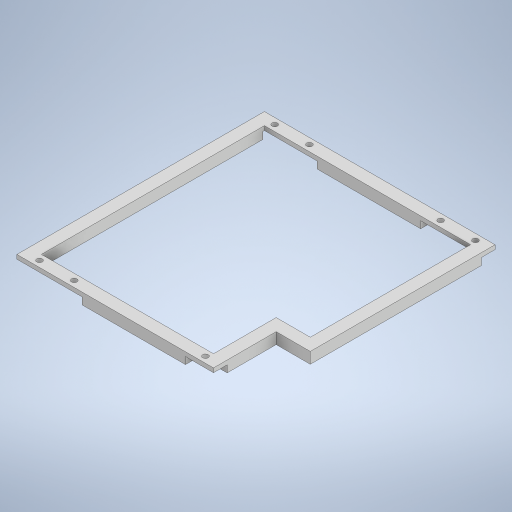
# Autodesk Inventor part: Base PCB
Saved by Autodesk Inventor 2024 (Build 280153000, 153)
## iProperties
Created: 2023-06-25
Part Number: Base PCB
Material: Genérico
Document SubType Name: Modeling
Designer: sergi
Density: 1 g/cm^3
Appearance: Valor por defecto
Author: sergi
Autodesk Inventor part; units mm, degrees
ref_plane "YZ Plane" through (0, 0, 0) normal (1, 0, 0) x (0, 1, 0)
ref_plane "XZ Plane" through (0, 0, 0) normal (0, 1, 0) x (-1, 0, 0)
ref_plane "XY Plane" through (0, 0, 0) normal (0, 0, 1) x (1, 0, 0)
sketch "Boceto1" plane through (0, 0, 0) normal (0, 1, 0) x (-1, 0, 0)
  line L0 (0, 0) -> (262.4667, 0) construction
  line L1 (262.4667, 0) -> (262.4667, -371.2633) construction
  line L2 (262.4667, -371.2633) -> (0, -371.2633) construction
  line L3 (0, -371.2633) -> (0, 0) construction
  line L4 (167.9771, -4.7349) -> (167.9771, -13.5349)
  line L5 (167.9771, -13.5349) -> (2.3545, -13.5349)
  line L6 (2.3545, -13.5349) -> (2.3545, -4.7349)
  line L7 (2.3545, -4.7349) -> (167.9771, -4.7349)
  line L8 (143.5689, -182.4039) -> (2.3545, -182.4039)
  line L9 (2.3545, -182.4039) -> (2.3545, -173.6039)
  line L10 (2.3545, -173.6039) -> (167.9771, -173.6039)
  line L11 (167.9771, -173.6039) -> (167.9771, -182.4039)
  circle A0 centre (156.1475, -9.1349) radius 2
  circle A1 centre (131.2333, -9.1349) radius 2
  circle A2 centre (12.066, -9.1349) radius 2
  line L12 (167.9771, -173.6039) -> (167.9771, -182.4039)
  line L13 (167.9771, -182.4039) -> (2.3545, -182.4039)
  line L14 (2.3545, -182.4039) -> (2.3545, -173.6039)
  line L15 (2.3545, -173.6039) -> (167.9771, -173.6039)
  circle A3 centre (131.2333, -178.0039) radius 2
  circle A4 centre (12.066, -178.0039) radius 2
  line L16 (167.9771, -13.5349) -> (167.9771, -182.4039)
  line L17 (2.3545, -13.4261) -> (2.3545, -174.0455)
  line L18 (11.1545, -13.4261) -> (11.1545, -174.0455)
  line L19 (159.1771, -13.5349) -> (159.1771, -182.4039)
  line L20 (26.8486, -4.7349) -> (26.8486, -49.7349)
  line L21 (26.8486, -49.7349) -> (2.3545, -49.7349)
  line L22 (35.6486, -4.7349) -> (35.6486, -58.5349)
  line L23 (35.6486, -58.5349) -> (2.3545, -58.5349)
  point P0 (11.1545, -173.6039)
  point P1 (11.1545, -13.5349)
  point P2 (159.1771, -173.6039)
  point P3 (11.1545, -58.5349)
  point P4 (35.6486, -13.5349)
  dimension "d2" = 8.8
  dimension "d3" = 8.8
  dimension "d5" = 8.8
  dimension "d6" = 8.8
  dimension "d8" = 4
  dimension "d9" = 4
  dimension "d10" = 4
  dimension "d11" = 8.8
  dimension "d12" = 8.8
  dimension "d14" = 4
  dimension "d15" = 4
  dimension "d21" = 8.8
  dimension "d22" = 8.8
  dimension "d26" = 45
  dimension "d27" = 8.8
  constraints: 40 end point, 8 perpendicular, 6 point on line, 5 centre point, 4 parallel, 2 vertical, 1 horizontal, 2 other
  measures "d2" distance of L4.start L4.end
  measures "d3" distance of L5.end L6.end
  measures "d5" distance of L8.end L9.end
  measures "d6" distance of L10.end L11.end
  measures "d8" diameter of A0
  measures "d9" diameter of A1
  measures "d10" diameter of A2
  measures "d11" distance of L12.start L13.start
  measures "d12" distance of L13.end L14.end
  measures "d14" diameter of A3
  measures "d15" diameter of A4
  measures "d21" distance between parallel lines of L17 L18
  measures "d22" distance between parallel lines of L16 L19
  measures "d26" distance of L20.start L20.end
  measures "d27" distance between parallel lines of L20 L22
extrude "Extrusión1" add sketch "Boceto1" along normal blind 3 contours L4 L5 L22 L7 | L16 L10 L19 L5 | L22 L5 L20 L7 | L11 L13 L19 L10 | L22 L23 L18 L21 L20 L5 | L19 L13 L8 L9 L10 | L10 L17 L23 L18 | L23 L17 L21 L18
sketch "Boceto2" plane through (0, 3, 0) normal (0, 1, 0) x (1, 0, 0)
  line L0 (-2.3545, 182.4039) -> (-167.9771, 182.4039) projected
  line L1 (-167.9771, 182.4039) -> (-167.9771, 4.7349) projected
  line L2 (-167.9771, 4.7349) -> (-26.8486, 4.7349) projected
  circle A0 centre (-12.066, 178.0039) radius 2
  circle A1 centre (-131.2333, 178.0039) radius 2
  circle A2 centre (-156.1475, 9.1349) radius 2
  circle A3 centre (-131.2333, 9.1349) radius 2
  line L3 (-11.1545, 173.6039) -> (-11.1545, 58.5349) projected
  line L4 (-35.6486, 13.5349) -> (-159.1771, 13.5349) projected
  line L5 (-159.1771, 13.5349) -> (-159.1771, 173.6039) projected
  line L6 (-159.1771, 173.6039) -> (-11.1545, 173.6039) projected
  line L7 (-131.2333, 9.1349) -> (-119.9333, 9.1349)
  line L8 (-119.9333, 9.1349) -> (-119.9333, 13.5349)
  line L9 (-119.9333, 4.7349) -> (-119.9333, 9.1349)
  line L10 (-167.9771, 4.7349) -> (-26.8486, 4.7349) projected
  line L11 (-26.8486, 4.7349) -> (-26.8486, 49.7349) projected
  line L12 (-26.8486, 49.7349) -> (-2.3545, 49.7349) projected
  line L13 (-2.3545, 49.7349) -> (-2.3545, 182.4039) projected
  line L14 (-11.1545, 58.5349) -> (-35.6486, 58.5349) projected
  line L15 (-35.6486, 58.5349) -> (-35.6486, 13.5349) projected
  circle A4 centre (-36.9802, 178.0039) radius 2
  circle A5 centre (-156.1475, 178.0039) radius 2
  circle A6 centre (-156.1475, 9.1349) radius 2
  line L16 (-156.1475, 9.1349) -> (-144.8475, 9.1349)
  line L17 (-144.8475, 9.1349) -> (-144.8475, 13.5349)
  line L18 (-144.8475, 4.7349) -> (-144.8475, 9.1349)
  line L19 (-36.9802, 178.0039) -> (-36.9802, 9.1349)
  line L20 (-36.9802, 178.0039) -> (131.8887, 178.0039) construction
  circle A7 centre (-36.9802, 9.1349) radius 2
  point P0 (0, 0)
  point P1 (-2.3545, 4.7349)
  dimension "d25" = 11.3
  dimension "d29" = 11.3
  dimension "d30" = 90
  dimension "d31" = 4
  constraints: 16 end point, 14 centre point, 3 perpendicular, 2 point on line, 1 coincident, 1 horizontal, 1 parallel
  measures "d25" distance of L7.start L7.end
  measures "d29" distance of L16.start L17.start
  measures "d30" angle of L19 L20
  measures "d31" diameter of A7
hole "Agujero1" at (-36.9802, 3, -9.1349) at (-36.9802, 3, -178.0039) at (-156.1475, 3, -178.0039) direction (0, -1, 0) diameter 4 end through all
sketch "Boceto3" plane through (0, 0, 0) normal (0, -1, 0) x (1, 0, 0)
  circle A0 centre (-156.1475, -178.0039) radius 2 projected
  circle A1 centre (-36.9802, -178.0039) radius 2 projected
  circle A2 centre (-36.9802, -9.1349) radius 2 projected
  line L0 (-167.9771, -182.4039) -> (-167.9771, -4.7349) projected
  line L1 (-2.3545, -182.4039) -> (-167.9771, -182.4039) projected
  line L2 (-2.3545, -49.7349) -> (-2.3545, -182.4039) projected
  line L3 (-26.8486, -49.7349) -> (-2.3545, -49.7349) projected
  line L4 (-26.8486, -4.7349) -> (-26.8486, -49.7349) projected
  line L5 (-167.9771, -4.7349) -> (-26.8486, -4.7349) projected
  circle A3 centre (-156.1475, -9.1349) radius 2 projected
  circle A4 centre (-131.2333, -9.1349) radius 2 projected
  line L6 (-159.1771, -173.6039) -> (-11.1545, -173.6039)
  line L7 (-159.1771, -13.5349) -> (-159.1771, -173.6039) projected
  line L8 (-35.6486, -13.5349) -> (-159.1771, -13.5349) projected
  line L9 (-35.6486, -58.5349) -> (-35.6486, -13.5349) projected
  line L10 (-11.1545, -58.5349) -> (-35.6486, -58.5349) projected
  line L11 (-11.1545, -173.6039) -> (-11.1545, -58.5349) projected
  circle A5 centre (-131.2333, -178.0039) radius 2 projected
  circle A6 centre (-12.066, -178.0039) radius 2 projected
  line L12 (-36.9802, -9.1349) -> (-46.9802, -9.1349)
  line L13 (-46.9802, -9.1349) -> (-46.9802, -2.3988)
  line L14 (-46.9802, -2.3988) -> (-46.9802, -182.4039)
  line L15 (-131.2333, -9.1349) -> (-121.2333, -9.1349)
  line L16 (-121.2333, -9.1349) -> (-121.2333, 4.8486)
  line L17 (-121.2333, 4.8486) -> (-121.2333, -182.4039)
  line L18 (-159.1771, -173.6039) -> (-167.9771, -173.6039)
  line L19 (-159.1771, -13.5349) -> (-167.9771, -13.5349)
  line L20 (-35.932, -13.5349) -> (-26.8486, -13.5349)
  line L21 (-11.1545, -173.6039) -> (-2.3545, -173.6039)
  line L22 (-2.3545, -172.6039) -> (-11.1545, -172.6039)
  line L23 (-11.1545, -172.6039) -> (-159.1771, -172.6039)
  line L24 (-159.1771, -172.6039) -> (-167.9771, -172.6039)
  line L25 (-35.932, -14.5349) -> (-26.8486, -14.5349)
  line L26 (-159.1771, -14.5349) -> (-167.9771, -14.5349)
  point P0 (0, 0)
  point P1 (-35.6486, -14.5349)
  point P2 (-121.2333, -173.6039)
  point P3 (-46.9802, -173.6039)
  point P4 (-121.2333, -13.5349)
  point P5 (-46.9802, -13.5349)
  point P6 (-46.9802, -4.7349)
  point P7 (-121.2333, -4.7349)
  dimension "d39" = 10
  dimension "d40" = 10
  dimension "d41" = 1
  dimension "d42" = 1
  dimension "d43" = 1
  constraints: 32 end point, 7 centre point, 6 point on line, 5 perpendicular, 3 parallel, 1 horizontal, 2 other
  measures "d39" distance of L12.start L12.end
  measures "d40" distance of L15.start L15.end
  measures "d41" distance between parallel lines of L21 L22
  measures "d42" distance between parallel lines of L20 L25
  measures "d43" distance between parallel lines of L19 L26
extrude "Extrusión2" add sketch "Boceto3" along normal blind 5 contours L17 L6 L14 L1 | L0 L26 L7 L24 | L17 L16 L5 L13 L14 L8 | L22 L11 L10 L9 L25 L4 L3 L2
